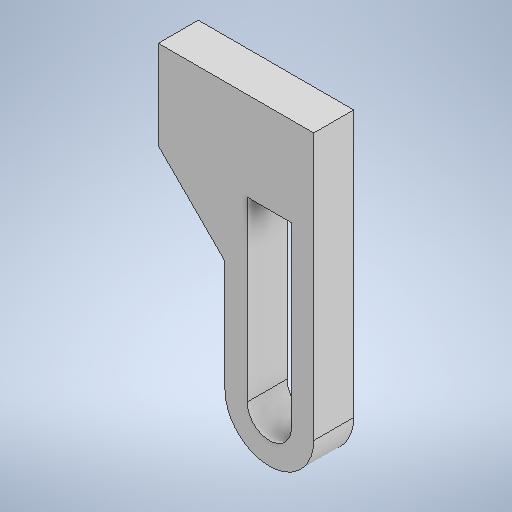
# Autodesk Inventor part: guide
Saved by Autodesk Inventor 2025.2 (Build 292293000, 293)
## iProperties
Created: 2025-02-15
Part Number: guide
Material: Generic
Document SubType Name: Modeling
Designer: kenne
Density: 1 g/cm^3
Appearance: Default
Author: kenne
Autodesk Inventor part; units mm, degrees
ref_plane "YZ Plane" through (0, 0, 0) normal (1, 0, 0) x (0, 1, 0)
ref_plane "XZ Plane" through (0, 0, 0) normal (0, 1, 0) x (-1, 0, 0)
ref_plane "XY Plane" through (0, 0, 0) normal (0, 0, 1) x (1, 0, 0)
sketch "Sketch1" plane through (0, 0, 0) normal (0, 0, 1) x (1, 0, 0)
  line L0 (0, 0) -> (0, 80) construction
  line L1 (0, 80) -> (10, 80) construction
  line L2 (0, 80) -> (-10, 80) construction
  line L3 (-10, 80) -> (10, 80)
  line L4 (10, 80) -> (10, 0)
  line L5 (-10, 80) -> (-10, 0)
  arc A0 (-10, 0) -> (10, 0) centre (0, 0) ccw
  line L6 (10, 0) -> (20, 0) construction
  line L7 (20, 0) -> (20, 120)
  line L8 (20, 120) -> (-50, 120)
  line L9 (-50, 120) -> (-50, 80)
  line L10 (-50, 120) -> (-20, 120) construction
  arc A1 (-20, 0) -> (20, 0) centre (0, 0) ccw
  line L11 (-20, 0) -> (-20, 50)
  line L12 (-20, 50) -> (-50, 80)
  dimension "d0" = 80
  dimension "d3" = 10
  dimension "d4" = 120
  dimension "d5" = 70
  dimension "d6" = 40
  dimension "d7" = 30
  dimension "d8" = 20
  dimension "d9" = 50
  constraints: 26 end point, 6 vertical, 4 horizontal, 4 point on circle, 2 centre point, 2 tangent, 1 collinear, 1 point on line
  measures "d0" distance of L0.start L0.end
  measures "d3" distance of L4.end L6.end
  measures "d4" distance of L6.end L7.end
  measures "d5" distance of L7.end L8.end
  measures "d6" distance of L8.end L9.end
  measures "d7" distance of L8.end L10.end
  measures "d8" radius of A1
  measures "d9" distance of L11.start L11.end
extrude "Extrusion1" add sketch "Sketch1" along normal blind 18
body "Solid1"
